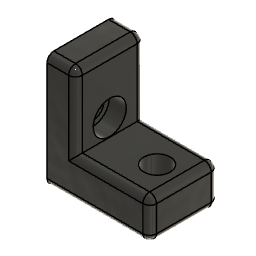
umbilical-mount (Autodesk Fusion 360 design; units mm, degrees)
Autodesk Fusion 360 part; units mm, degrees
sketch "Sketch1" plane through (0, 0, 0) normal (1, 0, 0) x (0, 1, 0)
  line L0 (142.8325, -5.8566) -> (154.8325, -5.8566)
  line L1 (154.8325, -5.8566) -> (154.8325, -25.8566)
  line L2 (142.8325, -5.8566) -> (142.8325, -25.8273)
  circle A0 centre (148.8325, -15.8566) radius 1.6
  circle A1 centre (148.8325, -15.8566) radius 2.9
  line L3 (142.8325, -25.8273) -> (154.8325, -25.8566)
  line L4 (154.8325, -25.8566) -> (142.8325, -25.8566)
  line L5 (142.8325, -25.8566) -> (142.8325, -18.8566)
  line L6 (142.8325, -18.8566) -> (154.8325, -18.8566)
  line L7 (154.8325, -18.8566) -> (154.8325, -25.8566)
  dimension "d64" = 12
  dimension "d65" = 20
  dimension "d71" = 3.2
  dimension "d72" = 5.8
  dimension "d73" = 6
  dimension "d74" = 10
  dimension "d158" = 7
  constraint horizontal L0
  constraint perpendicular L0 L1
  constraint perpendicular L0 L2
  constraint concentric A0 A1
  constraint horizontal L4
  constraint vertical L5
  constraint horizontal L6
  constraint vertical L7
  constraint coincident L2 L5.end
  measures "d64" distance of L0.start L0.end
  measures "d65" distance of L0.end L1.end
  measures "d71" diameter of A0
  measures "d72" diameter of A1
  measures "d73" distance of L1 A0.centre
  measures "d74" distance of L0 A0.centre
  measures "d158" distance of L4 L6
extrude "Extrude1" add sketch "Sketch1" against normal blind 1 contours L0 L1 L2 L6 | L1 L2 L3 L5 L6 L7 | A1 in component "MidPoint-Base"
extrude "Extrude2" add sketch "Sketch1" along normal blind 4 contours L0 L1 L2 L6 | L1 L2 L3 L5 L6 L7 in component "MidPoint-Base"
extrude "Extrude4" add sketch "Sketch1" along normal blind 1 contours A1 in component "MidPoint-Base"
sketch "Sketch2" plane through (-1, 0, 0) normal (-1, 0, 0) x (0, -1, 0)
  circle A0 centre (-148.8325, -15.8566) radius 1.6
  line L0 (-142.8325, -25.8273) -> (-142.8325, -5.8566)
  line L1 (-142.8325, -5.8566) -> (-154.8325, -5.8566)
  line L2 (-154.8325, -5.8566) -> (-154.8325, -25.8566)
  line L3 (-142.8325, -5.8566) -> (-154.8325, -5.8566)
  line L4 (-154.8325, -5.8566) -> (-154.8325, -25.8566)
  line L5 (-143.8325, -12.8566) -> (-153.8325, -12.8566)
  line L6 (-153.8325, -12.8566) -> (-153.8325, -18.8566)
  line L7 (-153.8325, -18.8566) -> (-143.8325, -18.8566)
  line L8 (-143.8325, -18.8566) -> (-143.8325, -12.8566)
  line L9 (-154.8325, -25.8566) -> (-142.8325, -25.8273)
  dimension "d142" = 1
  dimension "d143" = 1
  dimension "d144" = 7
  dimension "d145" = 6
  constraint horizontal L5
  constraint vertical L6
  constraint horizontal L7
  constraint vertical L8
  measures "d142" distance of L0 L8
  measures "d143" distance of L4 L6
  measures "d144" distance of L3 L5
  measures "d145" distance of L5 L7
extrude "Extrude5" add sketch "Sketch2" along normal blind 1.6 contours L5 L6 L7 L8 in component "MidPoint-Base"
extrude "Extrude7" add sketch "Sketch1" along normal blind 13 from surface at 4 contours L1 L2 L3 L5 L6 L7 in component "MidPoint-Base"
sketch "Sketch3" plane through (0, 0, -18.8566) normal (0, 0, 1) x (-1, 0, 0)
  line L0 (-4, -154.8325) -> (-4, -142.8325)
  line L1 (-4, -142.8325) -> (-17, -142.8325)
  line L2 (-17, -142.8325) -> (-17, -154.8325)
  line L3 (-17, -154.8325) -> (-4, -154.8325)
  circle A0 centre (-12.3, -148.8325) radius 2.3
  dimension "d153" = 4.6
  dimension "d154" = 12
  dimension "d155" = 6
  dimension "d159" = 8.3
  measures "d153" diameter of A0
  measures "d154" distance of L1 L3
  measures "d155" distance of L3 A0.centre
  measures "d159" distance of L0 A0.centre
extrude "Extrude8" cut sketch "Sketch3" against normal blind 6 contours A0 in component "MidPoint-Base"
chamfer "Chamfer3" distance 0.4 angle 45 1 edges at (1, 147.3408, -15.278) in component "MidPoint-Base"
fillet "Fillet2" radius 1.2 12 edges at (1.5, 154.8325, -5.8566) (4, 154.8325, -12.3566) (4, 148.8325, -5.8566) (4, 142.8325, -12.3566) (1.5, 142.8325, -5.8566) (10.5, 142.8325, -18.8566) (10.5, 154.8325, -18.8566) (17, 148.8325, -18.8566) (17, 154.8325, -22.3566) (8, 154.8325, -25.8566) (17, 148.8325, -25.842) (8, 142.8325, -25.8273) in component "MidPoint-Base"
fillet "Fillet2" radius 1.2 1 edges at (17, 142.8325, -22.342) in component "MidPoint-Base"
chamfer "Chamfer4" distance 0.6 distance2 1.2 2 edges at (-2.6, 148.8325, -18.8566) (-2.6, 148.8325, -12.8566) measured on face at (-2.6, 152.6992, -15.8566) measured on face at (-2.6, 152.6992, -15.8566) in component "MidPoint-Base"
chamfer "Chamfer4" distance 0.6 distance2 1.2 2 edges at (-2.6, 153.8325, -15.8566) (-2.6, 143.8325, -15.8566) measured on face at (-2.6, 152.6992, -15.8566) measured on face at (-2.6, 152.6992, -15.8566) in component "MidPoint-Base"
component "MidPoint-Base" placed x (1, 0, 0) y (0, 1, 0) z (0, 0, 1) at (0, 0, 0)
equation "d73 = d64 / 2"
equation "d142 = d143"
equation "d155 = 12.00 mm / 2"
equation "d159 = 6 mm + d153 / 2"
